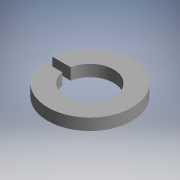
# Autodesk Inventor part: HCBST8_w1
Saved by Autodesk Inventor 2017.3 (Build 213256000, 256)
## iProperties
Part Number: HCBST8_w1
Material: Generic
Catalog Web Link: www.cadenas.de
Description: HCBST_washer1-Spring Washer Assembled Hexagon Socket Head Cap Screws
Vendor: MISUMI
Document SubType Name: Modeling
Designer: partserver
Manufacturer: MISUMI
Mass: 0.215477 g
Surface Area: 3.64999 cm^2
Volume: 0.215477 cm^3
Density: 1 g/cm^3
Appearance: PSOLRGB-192-192-192
Category: PARTsolutions
Company: MISUMI
Title: HCBST8
Author: Cadenas PARTsolutions
Comments: Spring Washer Assembled Hexagon Socket Head Cap Screws
PSOL_IDENT_0: {$CADENAS_DATA\23d-libs\misumi\metric\38_al_extrusions_blackets\nuts\hcbst_washer1.prj},163 {VTYP=3D
PSOL_IDENT_1: },{NB=HCBST8_w1},{LINA=HCBST8},{NN=HCBST_washer1},{DATE=17.06.2021 07:12:01},{GEOMDATE=15.04.2019 02
PSOL_IDENT_2: :23:09},{VERSION=},{LINEID=110},{WBVAR=},{WBNUMERIC=}  {NB=HCBST8_w1},{LINA=HCBST8},{KT=DUMMY},{PN=H
PSOL_IDENT_3: CBST8},{M=8},{M1=8},{MP=8x1.25},{P=1.250},{C=14.5},{D=17.0},{AA=8.4},{DD=8.2},{TT=2.0}
NB: HCBST8_w1
NN: HCBST_washer1
NT: Spring Washer Assembled Hexagon Socket Head Cap Screws
NBSYN: $PN._w1
LINA: HCBST8
CATALOG: Misumi
PN: HCBST8
M: 8
M1: 8
MP: 8x1.25
P: 1.25
C: 14.5
D: 17
AA: 8.4
DD: 8.2
TT: 2
SUPPLIER: MISUMI
ARTICLENO: HCBST8_w1
BOMINFO: HCBST8
CREATOR: CADENAS GmbH
Autodesk Inventor part; units mm, degrees
sketch "Sketch_1" plane through (0, 0, 0) normal (0, 0, 1) x (1, 0, 0)
  arc A0 (7.2137, 0.725) -> (7.2137, -0.725) centre (0, 0) ccw
  line L0 (7.2137, -0.725) -> (4.0354, -0.725)
  arc A1 (4.0354, 0.725) -> (4.0354, -0.725) centre (0, 0) ccw
  line L1 (4.0354, 0.725) -> (7.2137, 0.725)
  constraints: 4 end point, 4 point on circle, 2 centre point
extrude "Extrusion1" add sketch "Sketch_1" against normal blind 2
ref_plane "spring_washer_to_bolt_XY" through (0, 0, 0) normal (0, 0, 1) x (1, 0, 0)
ref_plane "spring_washer_to_bolt_YZ" through (0, 0, 0) normal (1, 0, 0) x (0, 1, 0)
ref_plane "spring_washer_to_bolt_ZX" through (0, 0, 0) normal (0, 1, 0) x (0, 0, 1)
ref_plane "spring_washer_to_washer_XY" through (0, 0, -2) normal (0, 0, 1) x (1, 0, 0)
ref_plane "spring_washer_to_washer_YZ" through (0, 0, -2) normal (1, 0, 0) x (0, 1, 0)
ref_plane "spring_washer_to_washer_ZX" through (0, 0, -2) normal (0, 1, 0) x (0, 0, 1)
body "Solid1"
